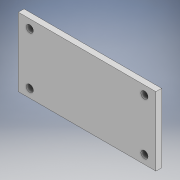
# Autodesk Inventor part: Arm Support Plate
Saved by Autodesk Inventor 2020 (Build 240168000, 168)
## iProperties
Created: 2019-10-01
Part Number: Arm Support Plate
Material: Generic
Document SubType Name: Modeling
Designer: Matt
Density: 1 g/cm^3
Appearance: Default
Author: Matt
Autodesk Inventor part; units mm, degrees
ref_plane "YZ Plane" through (0, 0, 0) normal (1, 0, 0) x (0, 1, 0)
ref_plane "XZ Plane" through (0, 0, 0) normal (0, 1, 0) x (-1, 0, 0)
ref_plane "XY Plane" through (0, 0, 0) normal (0, 0, 1) x (1, 0, 0)
sketch "Sketch1" plane through (0, 0, 0) normal (0, 0, 1) x (1, 0, 0)
  line L0 (-76.2, -38.1) -> (76.2, -38.1)
  line L1 (76.2, -38.1) -> (76.2, 38.1)
  line L2 (76.2, 38.1) -> (-76.2, 38.1)
  line L3 (-76.2, 38.1) -> (-76.2, -38.1)
  line L4 (-76.2, -38.1) -> (76.2, 38.1) construction
  line L5 (76.2, -38.1) -> (-76.2, 38.1) construction
  point P0 (0, 0)
  dimension "d0" = 152.4
  dimension "d1" = 76.2
  constraints: 12 end point, 2 midpoint, 2 parallel, 1 horizontal, 1 perpendicular
  measures "d0" distance of L2.end L1.end
  measures "d1" distance of L1.end L0.end
extrude "Extrusion1" add sketch "Sketch1" along normal blind 6.35
sketch "Sketch2" plane through (0, 0, 6.35) normal (0, 0, 1) x (1, 0, 0)
  line L0 (0, 0) -> (63.5, 0) construction
  line L1 (63.5, 0) -> (63.5, 28.575) construction
  line L2 (63.5, 28.575) -> (63.5, -28.575) construction
  line L3 (63.5, 28.575) -> (-63.5, 28.575) construction
  line L4 (-63.5, 28.575) -> (-63.5, -28.575) construction
  line L5 (-63.5, -28.575) -> (63.5, -28.575) construction
  line L6 (63.5, -28.575) -> (63.5, 28.575) construction
  dimension "d4" = 63.5
  dimension "d5" = 28.575
  dimension "d6" = 57.15
  dimension "d7" = 127
  dimension "d8" = 28.575
  constraints: 14 end point, 4 coincident, 2 horizontal, 2 parallel, 2 perpendicular, 1 point on line
  measures "d4" distance of L0.start L0.end
  measures "d5" distance of L0.end L1.end
  measures "d6" distance of L1.end L2.end
  measures "d7" distance of L5.end L4.end
  measures "d8" distance from line of L0.start L5
hole "Hole1" at (-63.5, 28.575, 6.35) at (-63.5, -28.575, 6.35) at (63.5, -28.575, 6.35) at (63.5, 28.575, 6.35) direction (0, 0, -1) diameter 7.9375 depth 19.05 tip angle 118
body "Solid1"
